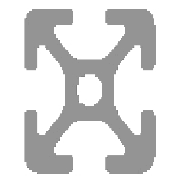
# Autodesk Inventor part: BT001_trajan20_22
Saved by Autodesk Inventor 2023 (Build 270158000, 158)
## iProperties
Created: 2022-10-30
Part Number: BT001_trajan20_22
Project: Zeichenmaschine_neu
Material: Generisch
Description: Bauteilname?
Document SubType Name: Modeling
Standard: item
Designer: Konstrukteur?
Language: de-DE
Size Designation: (Unbenannt 1)
Categories: <MemberInstance><Categories><Category DisplayName="Profile" InternalName="089c4875-fa83-4c05-b084-43b9cc11f5ed" Mnemonic="GRDR"><CategoryParameter DisplayName="Masse pro Längeneinheit" InternalName="0bb95a10-148f-4027-a459-38d7b056702a" Mnemonic="shpmass"/><CategoryParameter DisplayName="Querschnittsfläche" InternalName="1ff91680-64b0-4202-b9a3-7fd3f94bba3b" Mnemonic="secarea"/><CategoryParameter DisplayName="Trägheitsradius (x)" InternalName="25778675-03e9-40c1-b6a8-4a9ed693320d" Mnemonic="gyrradx"/><CategoryParameter DisplayName="Torsion-Festigkeitsmodul" InternalName="26c1ec35-5026-4c63-ad0a-751cf684a536" Mnemonic="torrigmod"/><CategoryParameter DisplayName="Abstand zum Schwerpunkt X-X" InternalName="26c9bdb8-9c79-4b4f-a92e-8e197583c9c4" Mnemonic="grcendistX"/><CategoryParameter DisplayName="Alte Varianten-ID" InternalName="340afe4f-75d7-48d3-ab7d-943f3c3da468" Mnemonic="LegacyMemberID"/><CategoryParameter DisplayName="Basislänge" InternalName="42e34263-8f20-4d0e-ad48-bf1385b87c24" Mnemonic="shplen"/><CategoryParameter DisplayName="Trägheitsmoment (y)" InternalName="4b9f58ea-bced-460e-81ea-3d29ca5a49e3" Mnemonic="inermomy"/><CategoryParameter DisplayName="Trägheitsmoment (x)" InternalName="4cd780bc-73d7-43ac-917a-579e5cbd684d" Mnemonic="inermomx"/><CategoryParameter DisplayName="Benutzerdefinierter Basispunkt" InternalName="4f1d1b73-316d-484b-a3df-9cbabb16eb77" Mnemonic="shpBasePoint"/><CategoryParameter DisplayName="Objekthöhe" InternalName="50274e7d-5ac0-4796-92cb-c59e54983c67" Mnemonic="shpheig"/><CategoryParameter DisplayName="Widerstandsmoment (y)" InternalName="59eaa5e9-d227-48dc-b6c1-6920f96e0f95" Mnemonic="secmody"/><CategoryParameter DisplayName="Schnittbezeichnung" InternalName="5a64d034-428d-49c8-ba32-7619764de20f" Mnemonic="shpdes"/><CategoryParameter DisplayName="Widerstandsmoment (x)" InternalName="72cfad18-cf51-4ed4-aaa7-c6b224f8419f" Mnemonic="secmodx"/><CategoryParameter DisplayName="Drehrissmodul" InternalName="7c55a8dc-8844-49f9-a867-cc677b30ec9a" Mnemonic="torsecmod"/><CategoryParameter DisplayName="Objektbreite" InternalName="7c717d54-a18f-4666-b4d4-573cce22c62c" Mnemonic="shpwdth"/><CategoryParameter DisplayName="Zweite Objektdicke" InternalName="9251a8e1-85fd-4e47-af99-afdb762317d9" Mnemonic="shpthick2"/><CategoryParameter DisplayName="GG Erstellt" InternalName="9c666724-f362-4ea7-ac62-f6a007de5c69" Mnemonic="shpFGAuto"/><CategoryParameter DisplayName="Abstand zum Schwerpunkt Y-Y" InternalName="bcc4fb17-7af4-436a-8f8c-d0aa3b0248c5" Mnemonic="grcendistY"/><CategoryParameter DisplayName="Trägheitsradius (y)" InternalName="bfa18ebe-1636-4dbe-8d42-b263e0b73184" Mnemonic="gyrrady"/><CategoryParameter DisplayName="Objektdicke" InternalName="d109cf76-8eb4-42fc-9800-4409734adc67" Mnemonic="shpthick"/><CategoryParameter DisplayName="Koeffizient für Schubverschiebung" InternalName="de4c90c6-aaa8-468f-a335-6737b311b5d3" Mnemonic="shdispc"/><Category DisplayName="Vierkantrohre (quadratisch/rechteckig)" InternalName="afc8e2d8-05d6-4609-8807-f98a9b7d2ed0" Mnemonic="SQRSHP"><CategoryParameter DisplayName="Querschnittsfläche" InternalName="2f7f79dd-983c-4263-802a-5b6a1495fdc5" Mnemonic="secarea"/><CategoryParameter DisplayName="Widerstandsmoment (x)" InternalName="50d965a6-04bf-46b9-8ace-861858d348e6" Mnemonic="secmodx"/><CategoryParameter DisplayName="Widerstandsmoment (y)" InternalName="5106aeac-54a2-4159-a9af-8933dd39dba2" Mnemonic="secmody"/><CategoryParameter DisplayName="Objektdicke" InternalName="52712fc5-f4ee-4eda-b3f2-6fce82c26419" Mnemonic="shpthick"/><CategoryParameter DisplayName="Trägheitsmoment (y)" InternalName="55ec8510-8276-4c45-8f10-594e0fee7eb3" Mnemonic="inermomy"/><CategoryParameter DisplayName="Trägheitsradius (x)" InternalName="56c89926-a299-4389-a862-ac94c9691272" Mnemonic="gyrradx"/><CategoryParameter DisplayName="Radius" InternalName="5d8d062c-e28e-41c1-98da-8e5fee36da1a" Mnemonic="shprad"/><CategoryParameter DisplayName="Trägheitsmoment (x)" InternalName="8c4637b6-6b69-4878-9d5d-26a32185d655" Mnemonic="inermomx"/><CategoryParameter DisplayName="Objektbreite" InternalName="8c8a1782-5e80-4d77-858b-304b1c0ad1fd" Mnemonic="shpwdth"/><CategoryParameter DisplayName="Trägheitsradius (y)" InternalName="fa48a7f5-f030-40f9-a60b-de8a845b7104" Mnemonic="gyrrady"/></Category></Category><Category DisplayName="Datentyp" InternalName="23b78d0f-2648-40c6-8793-ca6db495c9e8" Mnemonic="DATATYPE"><CategoryParameter DisplayName="Anzeigename" InternalName="05415f3d-3907-474b-a020-eb9d644f4cf3" Mnemonic="DISPLAYNAME"/><CategoryParameter DisplayName="Norm" InternalName="0c0a119c-1e12-4c84-803f-101930972f5e" Mnemonic="STANDARD"/><CategoryParameter DisplayName="Beschreibung" InternalName="13903e3d-64b1-4950-80da-f627842ea37f" Mnemonic="DESCRIPTION"/><CategoryParameter DisplayName="Bezeichnung" InternalName="2675968c-4ce5-49e0-a4f5-552d29089031" Mnemonic="DESIGNATION"/><CategoryParameter DisplayName="Standardzeile" InternalName="2af9ec52-faaa-4026-b378-f9fa4afca842" Mnemonic="DEFAULTROW"/><CategoryParameter DisplayName="Ordnername" InternalName="3f06958e-8713-4116-9be7-ed6184ecc97b" Mnemonic="FOLDERNAME"/><CategoryParameter DisplayName="Revisionsanleitung" InternalName="45a75005-10b1-4dfc-8d6d-dfe629f0b93c" Mnemonic="REVISIONGUID"/><CategoryParameter DisplayName="Dateiname" InternalName="8b46a4cc-9585-4fed-90c3-899f57e09a73" Mnemonic="FILENAME"/><CategoryParameter DisplayName="Normungsorganisation" InternalName="8f5914e1-4693-403f-8ab5-d37768198c9d" Mnemonic="STDSORG"/><CategoryParameter DisplayName="Gruppenversion" InternalName="914462f6-6e19-4b14-ba84-155b9680b1d0" Mnemonic="FAMILYREVISION"/><CategoryParameter DisplayName="Normrevision" InternalName="91d5a463-65c2-4fde-b823-3b7fea5e8e17" Mnemonic="STANDARDREVISION"/><CategoryParameter DisplayName="Variantenrevision" InternalName="a65d44b9-392f-4f4f-857b-e4b3d54996fe" Mnemonic="MEMBERREVISION"/><CategoryParameter DisplayName="ClipFormat" InternalName="bc51e27b-3422-4e78-93ef-cec197ddf230" Mnemonic="CLIPFORMAT"/><CategoryParameter DisplayName="Hersteller" InternalName="cd6c7a72-a28a-4e50-99a9-2c7f4e13e5ad" Mnemonic="MANUFACTURER"/><CategoryParameter DisplayName="InternerName" InternalName="cf1d0246-76d9-4b4a-8305-fa0409afb5c1" Mnemonic="INTERNALNAME"/><CategoryParameter DisplayName="IstMetrisch" InternalName="e2385c5b-1ea4-4823-96a8-8de651266ec3" Mnemonic="ISMETRIC"/><Category DisplayName="Bauteil" InternalName="c0e0b642-3bcb-4cc8-9e80-f96d35c4afa4" Mnemonic="PART"><CategoryParameter DisplayName="Bauteilnummer" InternalName="016b6077-bfbe-49bd-92c9-d8d59c39c941" Mnemonic="PARTNUMBER"/><CategoryParameter DisplayName="Bestandsnummer" InternalName="4dba7c1c-e26c-444e-836c-b08b433409a8" Mnemonic="STOCKNUMBER"/><CategoryParameter DisplayName="Materialschlüssel" InternalName="5c9a8adb-dd2b-4535-b97f-0a94a95fe41f" Mnemonic="MATERIALKEY"/><CategoryParameter DisplayName="Material" InternalName="818a152a-d3c3-49ca-80ee-df7d91421b8e" Mnemonic="MATERIAL"/></Category></Category></Categories><FamilyTemplate Id="BT001_trajan20_22_Zeichenmaschine_neu_item_20x20x5_ohne_Endbearbeitungen"><FamilyTemplateParameters><FamilyTemplateParameter ObjectType="kModelParameterObject" ValueType="xs:double" Id="12" ObjectReferenceKey="B_L"/><FamilyTemplateParameter ObjectType="kPartComponentDefinitionObject" ValueType="xs:string" Id="23" SubObjectId="Material"/><FamilyTemplateParameter ObjectType="kPropertyObject" ValueType="xs:string" Id="26" ObjectReferenceKey="{32853F0F-3444-11d1-9E93-0060B03C1CA6}" SubObjectId="5"/><FamilyTemplateParameter ObjectType="kPropertyObject" ValueType="xs:string" Id="27" ObjectReferenceKey="{32853F0F-3444-11d1-9E93-0060B03C1CA6}" SubObjectId="52"/></FamilyTemplateParameters></FamilyTemplate><CategoryParameterMap><ParamToTemplateMap><ParamToTemplate CategoryParameter="//CategoryParameter[@InternalName='cf1d0246-76d9-4b4a-8305-fa0409afb5c1']" ConstantValue="98368311-0f25-47e1-bf33-b5830556ecfc"/><ParamToTemplate CategoryParameter="//CategoryParameter[@InternalName='45a75005-10b1-4dfc-8d6d-dfe629f0b93c']" ConstantValue="a7594c96-df73-4dfc-bd75-cb8bb44b9089"/><ParamToTemplate CategoryParameter="//CategoryParameter[@InternalName='3f06958e-8713-4116-9be7-ed6184ecc97b']" ConstantValue="20x20x5_ohne_Endbearbeitungen"/><ParamToTemplate CategoryParameter="//CategoryParameter[@InternalName='8f5914e1-4693-403f-8ab5-d37768198c9d']" TemplateParameter="17"/><ParamToTemplate CategoryParameter="//CategoryParameter[@InternalName='0c0a119c-1e12-4c84-803f-101930972f5e']" ConstantValue="item"/><ParamToTemplate CategoryParameter="//CategoryParameter[@InternalName='91d5a463-65c2-4fde-b823-3b7fea5e8e17']" TemplateParameter="19"/><ParamToTemplate CategoryParameter="//CategoryParameter[@InternalName='cd6c7a72-a28a-4e50-99a9-2c7f4e13e5ad']" TemplateParameter="20"/><ParamToTemplate CategoryParameter="//CategoryParameter[@InternalName='13903e3d-64b1-4950-80da-f627842ea37f']" ConstantValue="item_20x20x5_ohne_Endbearbeitungen"/><ParamToTemplate CategoryParameter="//CategoryParameter[@InternalName='05415f3d-3907-474b-a020-eb9d644f4cf3']" ConstantValue="20x20x5_ohne_Endbearbeitungen"/><ParamToTemplate CategoryParameter="//CategoryParameter[@InternalName='914462f6-6e19-4b14-ba84-155b9680b1d0']" ConstantValue="11"/><ParamToTemplate CategoryParameter="//CategoryParameter[@InternalName='bc51e27b-3422-4e78-93ef-cec197ddf230']" ConstantValue="CF_INVENTOR.STDPARTS"/><ParamToTemplate CategoryParameter="//CategoryParameter[@InternalName='e2385c5b-1ea4-4823-96a8-8de651266ec3']" ConstantValue="true"/><ParamToTemplate CategoryParameter="//CategoryParameter[@InternalName='2af9ec52-faaa-4026-b378-f9fa4afca842']" ConstantValue="1"/><ParamToTemplate CategoryParameter="//CategoryParameter[@InternalName='9c666724-f362-4ea7-ac62-f6a007de5c69']" ConstantValue="1"/><ParamToTemplate CategoryParameter="//CategoryParameter[@InternalName='8b46a4cc-9585-4fed-90c3-899f57e09a73']" ConstantValue="50"/><ParamToTemplate CategoryParameter="//CategoryParameter[@InternalName='a65d44b9-392f-4f4f-857b-e4b3d54996fe']" ConstantValue="65b9e0b3-773f-4eb7-b09a-a0a309a4aeaf"/><ParamToTemplate CategoryParameter="//CategoryParameter[@InternalName='a65d44b9-392f-4f4f-857b-e4b3d54996fe']" ConstantValue="65b9e0b3-773f-4eb7-b09a-a0a309a4aeaf"/><ParamToTemplate CategoryParameter="//CategoryParameter[@InternalName='42e34263-8f20-4d0e-ad48-bf1385b87c24']" TemplateParameter="12"/><ParamToTemplate CategoryParameter="//CategoryParameter[@InternalName='2675968c-4ce5-49e0-a4f5-552d29089031']" TemplateParameter="27"/><ParamToTemplate CategoryParameter="//CategoryParameter[@InternalName='818a152a-d3c3-49ca-80ee-df7d91421b8e']" TemplateParameter="23"/><ParamToTemplate CategoryParameter="//CategoryParameter[@InternalName='016b6077-bfbe-49bd-92c9-d8d59c39c941']" TemplateParameter="26"/></ParamToTemplateMap></CategoryParameterMap></MemberInstance>
Mass: 22.0622 g
Surface Area: 206.615 cm^2
Volume: 22.0622 cm^3
Density: 1 g/cm^3
Appearance: Vorgabe
Company: HTBLA Kaindorf
RuleStatus: InUse
AfterDocNew0: iProperties-Editor_aufrufen
G_L: 120,000 mm
G_W: 20,000 mm
G_H: 20,000 mm
IsCustomPart: 1
_CCFamilyDisplayName: 20x20x5_ohne_Endbearbeitungen - item_20x20x5_ohne_Endbearbeitungen
_FrameMemberDoc: Frame Member File
_Version: 15.0.0
_GetPNFromCC: 1
Author: jan
Keywords: Schuljahr?
Autodesk Inventor part; units mm, degrees
ref_plane "YZ Plane" through (0, 0, 0) normal (1, 0, 0) x (0, 1, 0)
ref_plane "Startebene" through (0, 0, 0) normal (0, 0, 1) x (1, 0, 0)
ref_plane "Endebene" through (0, 0, 120) normal (0, 0, 1) x (1, 0, 0)
sketch "Skizze" plane through (0, 0, 0) normal (0, 0, 1) x (1, 0, 0)
  arc A0 (-4.5287, -3.2559) -> (-3.65, -1.1346) centre (-6.65, -1.1346) ccw
  line L0 (-3.65, -1.1346) -> (-3.65, 1.1346)
  circle A1 centre (0, 0) radius 2.15
  line L1 (1.1346, -3.65) -> (-1.1346, -3.65)
  arc A2 (-1.1346, -3.65) -> (-3.2559, -4.5287) centre (-1.1346, -6.65) ccw
  line L2 (-6.779, -5.5062) -> (-4.5287, -3.2559)
  line L3 (-3.2559, -4.5287) -> (-5.5062, -6.779)
  arc A3 (-2.5, -8.5) -> (-2.8, -8.2) centre (-2.8, -8.5) ccw
  line L4 (-2.5, -8.5) -> (-2.5, -9.2)
  line L5 (-4.9176, -8.2) -> (-2.8, -8.2)
  arc A4 (-5.5062, -6.779) -> (-4.9176, -8.2) centre (-4.9176, -7.3676) ccw
  arc A5 (-3.3, -10) -> (-2.5, -9.2) centre (-3.3, -9.2) ccw
  line L6 (-3.3, -10) -> (-8, -10)
  line L7 (10, -3.3) -> (10, -8)
  line L8 (5.5062, -6.779) -> (3.2559, -4.5287)
  arc A6 (6.779, -5.5062) -> (8.2, -4.9176) centre (7.3676, -4.9176) ccw
  arc A7 (3.2559, -4.5287) -> (1.1346, -3.65) centre (1.1346, -6.65) ccw
  line L9 (4.5287, -3.2559) -> (6.779, -5.5062)
  arc A8 (3.65, -1.1346) -> (4.5287, -3.2559) centre (6.65, -1.1346) ccw
  arc A9 (8.5, -2.5) -> (8.2, -2.8) centre (8.5, -2.8) ccw
  line L10 (3.65, 1.1346) -> (3.65, -1.1346)
  line L11 (8.5, -2.5) -> (9.2, -2.5)
  arc A10 (10, -3.3) -> (9.2, -2.5) centre (9.2, -3.3) ccw
  line L12 (8.2, -4.9176) -> (8.2, -2.8)
  line L13 (2.5, 8.5) -> (2.5, 9.2)
  arc A11 (2.5, 8.5) -> (2.8, 8.2) centre (2.8, 8.5) ccw
  arc A12 (1.1346, 3.65) -> (3.2559, 4.5287) centre (1.1346, 6.65) ccw
  line L14 (-1.1346, 3.65) -> (1.1346, 3.65)
  arc A13 (3.3, 10) -> (2.5, 9.2) centre (3.3, 9.2) ccw
  line L15 (4.9176, 8.2) -> (2.8, 8.2)
  arc A14 (4.5287, 3.2559) -> (3.65, 1.1346) centre (6.65, 1.1346) ccw
  line L16 (3.2559, 4.5287) -> (5.5062, 6.779)
  arc A15 (5.5062, 6.779) -> (4.9176, 8.2) centre (4.9176, 7.3676) ccw
  line L17 (6.779, 5.5062) -> (4.5287, 3.2559)
  line L18 (3.3, 10) -> (8, 10)
  arc A16 (10, 8) -> (8, 10) centre (8, 8) ccw
  line L19 (8.2, 2.8) -> (8.2, 4.9176)
  line L20 (10, 8) -> (10, 3.3)
  arc A17 (8.2, 4.9176) -> (6.779, 5.5062) centre (7.3676, 4.9176) ccw
  line L21 (-2.8, 8.2) -> (-4.9176, 8.2)
  line L22 (-2.5, 9.2) -> (-2.5, 8.5)
  arc A18 (-2.5, 9.2) -> (-3.3, 10) centre (-3.3, 9.2) ccw
  arc A19 (-2.8, 8.2) -> (-2.5, 8.5) centre (-2.8, 8.5) ccw
  arc A20 (-3.65, 1.1346) -> (-4.5287, 3.2559) centre (-6.65, 1.1346) ccw
  arc A21 (-3.2559, 4.5287) -> (-1.1346, 3.65) centre (-1.1346, 6.65) ccw
  arc A22 (4.9176, -8.2) -> (5.5062, -6.779) centre (4.9176, -7.3676) ccw
  arc A23 (8, -10) -> (10, -8) centre (8, -8) ccw
  line L23 (2.8, -8.2) -> (4.9176, -8.2)
  line L24 (8, -10) -> (3.3, -10)
  arc A24 (2.8, -8.2) -> (2.5, -8.5) centre (2.8, -8.5) ccw
  arc A25 (2.5, -9.2) -> (3.3, -10) centre (3.3, -9.2) ccw
  line L25 (2.5, -9.2) -> (2.5, -8.5)
  arc A26 (8.2, 2.8) -> (8.5, 2.5) centre (8.5, 2.8) ccw
  line L26 (9.2, 2.5) -> (8.5, 2.5)
  arc A27 (9.2, 2.5) -> (10, 3.3) centre (9.2, 3.3) ccw
  arc A28 (-4.9176, 8.2) -> (-5.5062, 6.779) centre (-4.9176, 7.3676) ccw
  line L27 (-8, 10) -> (-3.3, 10)
  line L28 (-5.5062, 6.779) -> (-3.2559, 4.5287)
  arc A29 (-8, 10) -> (-10, 8) centre (-8, 8) ccw
  arc A30 (-6.779, 5.5062) -> (-8.2, 4.9176) centre (-7.3676, 4.9176) ccw
  line L29 (-10, 3.3) -> (-10, 8)
  line L30 (-8.2, 4.9176) -> (-8.2, 2.8)
  arc A31 (-8.5, 2.5) -> (-8.2, 2.8) centre (-8.5, 2.8) ccw
  line L31 (-8.5, 2.5) -> (-9.2, 2.5)
  arc A32 (-10, 3.3) -> (-9.2, 2.5) centre (-9.2, 3.3) ccw
  line L32 (-4.5287, 3.2559) -> (-6.779, 5.5062)
  line L33 (-10, -8) -> (-10, -3.3)
  arc A33 (-8.2, -4.9176) -> (-6.779, -5.5062) centre (-7.3676, -4.9176) ccw
  arc A34 (-10, -8) -> (-8, -10) centre (-8, -8) ccw
  line L34 (-10, -8) -> (-10, -3.3)
  arc A35 (-8.2, -2.8) -> (-8.5, -2.5) centre (-8.5, -2.8) ccw
  line L35 (-9.2, -2.5) -> (-8.5, -2.5)
  arc A36 (-9.2, -2.5) -> (-10, -3.3) centre (-9.2, -3.3) ccw
  line L36 (-8.2, -2.8) -> (-8.2, -4.9176)
  dimension "d4" = 4.3
  dimension "d5" = 6.35
  dimension "d6" = 10
  dimension "d7" = 2.5
  dimension "d8" = 5.8
  dimension "d9" = 10.5
  dimension "d10" = 3
  dimension "d11" = 7.5
  dimension "d12" = 12.5
  dimension "d13" = 13.65
  dimension "d14" = 5.7
  dimension "d15" = 10.7
  dimension "d16" = 1.15
  dimension "d17" = 6.15
  dimension "d18" = 1.8
  dimension "d19" = 0.8
  dimension "d20" = 0.3
  dimension "d21" = 2
  dimension "d22" = 0.8324
  dimension "d23" = 45
  dimension "d24" = 90
  dimension "d25" = 90
  dimension "d26" = 1.8
  dimension "d27" = 18.2
  dimension "d28" = 20
  dimension "d29" = 5
  dimension "d30" = 7.5
  dimension "d31" = 1.8
  dimension "d32" = 0.9
  dimension "d33" = 0.9
  dimension "d34" = 20
  constraints: 102 tangent, 74 end point, 72 point on circle, 37 centre point, 31 equal radius, 18 parallel, 2 coincident, 1 horizontal, 1 perpendicular, 1 vertical
  measures "d4" diameter of A1
  measures "d5" distance between parallel lines of L20 L10
  measures "d6" distance from line of A1.centre L20
  measures "d7" distance from line of A1.centre L26
  measures "d8" distance from line of L33.end L26
  measures "d9" distance from line of L33.start L26
  measures "d10" radius of A14
  measures "d11" distance between parallel lines of L20 L13
  measures "d12" distance between parallel lines of L20 L22
  measures "d13" distance between parallel lines of L20 L0
  measures "d14" distance between parallel lines of L15 L26
  measures "d15" distance between parallel lines of L23 L26
  measures "d16" distance between parallel lines of L14 L26
  measures "d17" distance between parallel lines of L1 L26
  measures "d18" distance between parallel lines of L9 L8
  measures "d19" radius of A27
  measures "d20" radius of A26
  measures "d21" radius of A16
  measures "d22" radius of A17
  measures "d23" angle of L17 L20
  measures "d24" angle of L12 L26
  measures "d25" angle of L36 L26
  measures "d26" distance between parallel lines of L20 L19
  measures "d27" distance between parallel lines of L20 L30
  measures "d28" distance between parallel lines of L33 L20
  measures "d29" distance between parallel lines of L11 L26
  measures "d30" distance between parallel lines of L18 L26
  measures "d31" distance between parallel lines of L17 L16
  measures "d32" distance from line of point (0, 0) L17
  measures "d33" distance from line of point (0, 0) L9
  measures "d34" distance between parallel lines of L24 L18
extrude "Körper" add sketch "Skizze" along normal up to surface (120 mm away) from surface at 0
sketch "Skizze6" plane through (0, 0, 0) normal (0, 0, 1) x (1, 0, 0)
  line L0 (0, 0) -> (10, 0)
ref_plane "Arbeitsebene4" through (0, 0, 0) normal (0, -1, 0) x (1, 0, 0)
sketch "Skizze7" plane through (0, 0, 0) normal (0, -1, 0) x (1, 0, 0)
  line L0 (-2, 0) -> (12, 0)
  line L1 (-2, 120) -> (12, 120)
  dimension "d43" = 120
  measures "d43" distance between parallel lines of L0 L1
equation "\"G_OFFSET_START\" = 0"
equation "\"G_OFFSET_END\" = 0"
equation "\"G_L\" = d43"
